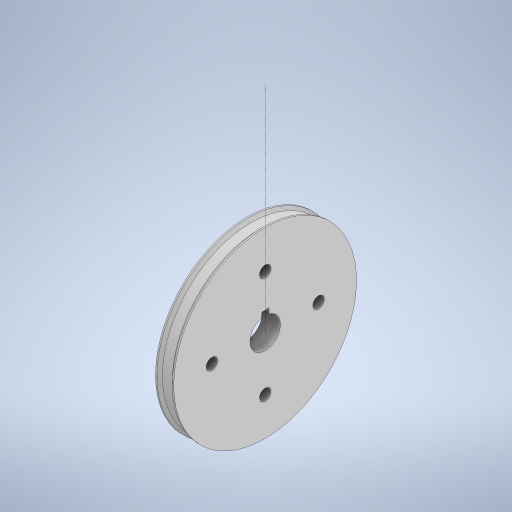
# Autodesk Inventor part: P#2_LAB_DINAMICA
Saved by Autodesk Inventor 2024 (Build 280153000, 153)
## iProperties
Created: 2024-02-19
Part Number: P#2_LAB_DINAMICA
Material: Generic
Document SubType Name: Modeling
Designer: aacas
Density: 1 g/cm^3
Appearance: Default
Author: aacas
Autodesk Inventor part; units mm, degrees
ref_plane "YZ Plane" through (0, 0, 0) normal (1, 0, 0) x (0, 1, 0)
ref_plane "XZ Plane" through (0, 0, 0) normal (0, 1, 0) x (-1, 0, 0)
ref_plane "XY Plane" through (0, 0, 0) normal (0, 0, 1) x (1, 0, 0)
sketch "Sketch1" plane through (0, 0, 0) normal (0, 0, 1) x (1, 0, 0)
  line L0 (0, 0) -> (-120, 0)
  line L1 (-120, 0) -> (-120, 600)
  line L2 (0, 600) -> (0, 0)
  line L3 (-120, 600) -> (-110, 600)
  line L4 (0, 600) -> (-10, 600)
  line L5 (-60, 582.32) -> (-27.68, 582.32)
  line L6 (-60, 582.32) -> (-92.32, 582.32)
  line L7 (-110, 600) -> (-92.32, 582.32)
  line L8 (-27.68, 582.32) -> (-10, 600)
  line L9 (-120, 600) -> (-110, 600)
  line L10 (-10, 600) -> (0, 600)
  dimension "d0" = 120
  dimension "d1" = 600
  dimension "d3" = 10
  dimension "d4" = 10
  dimension "d5" = 32.32
  dimension "d6" = 32.32
  constraints: 22 end point, 3 horizontal, 3 parallel, 1 perpendicular
  measures "d0" distance of L1.end L2.start
  measures "d1" distance of L0.end L1.end
  measures "d3" distance of L1.end L3.end
  measures "d4" distance of L2.start L4.end
  measures "d5" distance of L5.start L5.end
  measures "d6" distance of L5.start L6.end
sketch "Sketch2" plane through (0, 0, 0) normal (1, 0, 0) x (0, 1, 0)
  circle A0 centre (0, 0) radius 100
  dimension "d7" = 200
  constraints: 1 centre point, 1 coincident
  measures "d7" diameter of A0
sketch "Sketch3" plane through (0, 0, 0) normal (0, 0, 1) x (1, 0, 0)
  line L0 (0, 0) -> (0, 1416.3001) construction
  constraints: 2 end point, 1 vertical
revolve "Revolution1" add sketch "Sketch1" angle 360 about axis through (0, 0, 0) along (-1, 0, 0)
extrude "Extrusion1" cut sketch "Sketch2" against normal through all
sketch "Sketch4" plane through (0, 0, 0) normal (1, 0, 0) x (0, 0, -1)
  circle A0 centre (0, 0) radius 100 projected
  line L0 (0, 0) -> (25, 0)
  line L1 (25, 96.8246) -> (25, 130)
  line L2 (25, 130) -> (0, 130)
  line L3 (0, 0) -> (-26.4239, 0)
  line L4 (-26.4239, 96.4457) -> (-26.4239, 130)
  line L5 (-26.4239, 130) -> (0, 130)
  dimension "d11" = 25
  dimension "d12" = 130
  constraints: 12 end point, 2 horizontal, 2 parallel, 2 perpendicular, 2 point on circle
  measures "d11" distance of L2.end L1.end
  measures "d12" distance of L1.end L0.end
extrude "Extrusion2" cut sketch "Sketch4" against normal through all contours A0 L4 L5 L2 L1
sketch "Sketch5" plane through (0, 0, 0) normal (1, 0, 0) x (0, 0, -1)
  line L0 (0, 0) -> (350, 0)
  line L1 (0, 0) -> (0, 350)
  line L2 (0, 0) -> (-350, 0)
  line L3 (0, 0) -> (0, -350)
  circle A0 centre (0, 350) radius 37.5
  circle A1 centre (350, 0) radius 37.5
  circle A2 centre (0, -350) radius 37.5
  circle A3 centre (-350, 0) radius 37.5
  dimension "d15" = 350
  dimension "d16" = 350
  dimension "d17" = 350
  dimension "d18" = 350
  dimension "d19" = 75
  dimension "d20" = 75
  dimension "d21" = 75
  dimension "d22" = 75
  constraints: 8 end point, 4 centre point, 4 coincident, 2 horizontal, 1 perpendicular, 1 vertical
  measures "d15" distance of L0.start L0.end
  measures "d16" distance of L0.start L1.end
  measures "d17" distance of L0.start L2.end
  measures "d18" distance of L0.start L3.end
  measures "d19" diameter of A0
  measures "d20" diameter of A1
  measures "d21" diameter of A2
  measures "d22" diameter of A3
extrude "Extrusion3" cut sketch "Sketch5" against normal through all
body "Solid1"
